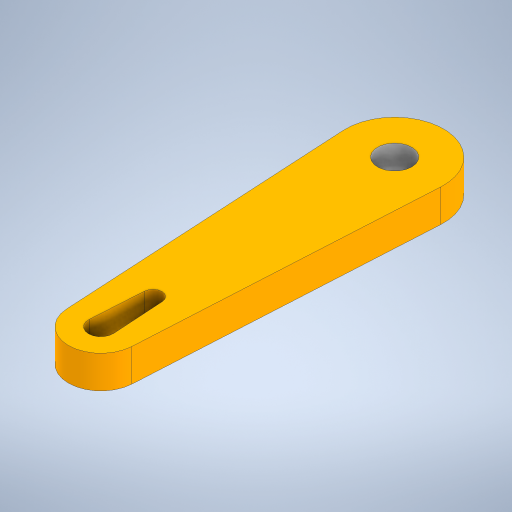
# Autodesk Inventor part: Brazo
Saved by Autodesk Inventor 2024 (Build 280153000, 153)
## iProperties
Created: 2024-04-28
Part Number: Brazo
Material: Generic
Document SubType Name: Modeling
Designer: samue
Density: 1 g/cm^3
Appearance: Default
Author: samue
Autodesk Inventor part; units mm, degrees
ref_plane "YZ Plane" through (0, 0, 0) normal (1, 0, 0) x (0, 1, 0)
ref_plane "XZ Plane" through (0, 0, 0) normal (0, 1, 0) x (-1, 0, 0)
ref_plane "XY Plane" through (0, 0, 0) normal (0, 0, 1) x (1, 0, 0)
sketch "Sketch1" plane through (0, 0, 0) normal (0, 1, 0) x (-1, 0, 0)
  circle A0 centre (-0.0087, 99.7911) radius 10
  circle A1 centre (-0.0022, 9.7911) radius 15
  line L0 (9.9759, 100.3474) -> (14.9746, 10.6255)
  line L1 (-9.9933, 100.346) -> (-14.9791, 10.6234)
  point P0 (0, 0)
  dimension "d0" = 20
  dimension "d1" = 30
  dimension "d2" = 90
  constraints: 4 end point, 4 point on circle, 4 tangent, 2 centre point
  measures "d0" diameter of A0
  measures "d1" diameter of A1
  measures "d2" distance of A1.centre A0.centre
extrude "Extrusion1" add sketch "Sketch1" against normal blind 10
sketch "Sketch2" plane through (0, 0, 0) normal (0, 1, 0) x (1, 0, 0)
  circle A0 centre (0, -99.8683) radius 3.75
  circle A1 centre (0, -83.8683) radius 2.75
  line L0 (2.7446, -83.6964) -> (3.7427, -99.6339)
  line L1 (-3.7427, -99.6339) -> (-2.7446, -83.6964)
  point P0 (0, 0)
  dimension "d7" = 7.5
  dimension "d8" = 5.5
  dimension "d9" = 16
  constraints: 4 end point, 4 point on circle, 4 tangent, 2 centre point
  measures "d7" diameter of A0
  measures "d8" diameter of A1
  measures "d9" distance of A0.centre A1.centre
extrude "Extrusion2" cut sketch "Sketch2" against normal blind 8.5
sketch "Sketch3" plane through (0, -8.5, 0) normal (0, 1, 0) x (1, 0, 0)
  arc A0 (-3.7427, -99.6339) -> (3.7427, -99.6339) centre (0, -99.8683) ccw projected
  circle A1 centre (0, -99.8683) radius 3.65
  point P0 (0, 0)
  dimension "d12" = 7.3
  constraints: 1 centre point, 1 coincident
  measures "d12" diameter of A1
extrude "Extrusion3" cut sketch "Sketch3" against normal blind 8.5
sketch "Sketch4" plane through (0, 0, 0) normal (0, 1, 0) x (1, 0, 0)
  arc A0 (14.9791, -10.6234) -> (-14.9746, -10.6255) centre (0.0022, -9.7911) ccw projected
  circle A1 centre (0.0022, -9.7911) radius 5.25
  point P0 (0, 0)
  dimension "d15" = 10.5
  constraints: 1 centre point, 1 coincident
  measures "d15" diameter of A1
extrude "Extrusion4" cut sketch "Sketch4" against normal blind 11
body "Solid1"
